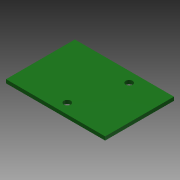
# Autodesk Inventor part: AmpPSBoard
Saved by Autodesk Inventor 2014 (Build 180170000, 170)
## iProperties
Created: 2015-04-19
Part Number: AmpPSBoard
Material: Generic
Document SubType Name: Modeling
Designer: Owner
Density: 1 g/cm^3
Appearance: Smooth - Dark Forest Green
Author: Owner
Autodesk Inventor part; units mm, degrees
ref_plane "YZ Plane" through (0, 0, 0) normal (1, 0, 0) x (0, 1, 0)
ref_plane "XZ Plane" through (0, 0, 0) normal (0, 1, 0) x (-1, 0, 0)
ref_plane "XY Plane" through (0, 0, 0) normal (0, 0, 1) x (1, 0, 0)
sketch "Sketch1" plane through (0, 0, 0) normal (0, 1, 0) x (-1, 0, 0)
  line L0 (-23.7026, 13.2984) -> (22.0174, 13.2984)
  line L1 (22.0174, 13.2984) -> (22.0174, -18.4516)
  line L2 (22.0174, -18.4516) -> (-23.7026, -18.4516)
  line L3 (-23.7026, -18.4516) -> (-23.7026, 13.2984)
  point P0 (0, 0)
  dimension "d0" = 45.72
  dimension "d1" = 31.75
  constraints: 8 end point, 2 parallel, 1 horizontal, 1 perpendicular
  measures "d0" distance of L0.start L0.end
  measures "d1" distance of L0.end L1.end
extrude "Extrusion1" add sketch "Sketch1" along normal blind 1.65
sketch "Sketch2" plane through (0, 1.65, 0) normal (0, 1, 0) x (1, 0, 0)
  line L0 (-22.0174, -13.2984) -> (23.7026, -13.2984) projected
  line L1 (23.7026, -13.2984) -> (23.7026, 18.4516) projected
  line L2 (23.7026, 18.4516) -> (-22.0174, 18.4516) projected
  circle A0 centre (1.4776, -8.5359) radius 1.5875
  circle A1 centre (7.8276, 13.6891) radius 1.5875
  point P0 (0, 0)
  dimension "d4" = 3.175
  dimension "d5" = 3.175
  dimension "d6" = 4.7625
  dimension "d7" = 4.7625
  dimension "d10" = 15.875
  dimension "d11" = 22.225
  constraints: 2 centre point
  measures "d4" diameter of A1
  measures "d5" diameter of A0
  measures "d6" distance from line of L0 A0.centre
  measures "d7" distance from line of L2 A1.centre
  measures "d10" distance from line of L1 A1.centre
  measures "d11" distance from line of L1 A0.centre
extrude "Extrusion2" cut sketch "Sketch2" against normal up to next
body "Solid1"
